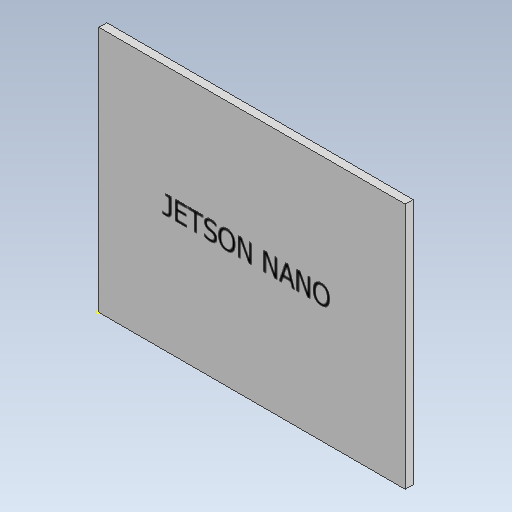
# Autodesk Inventor part: jetson_nano_sketch
Saved by Autodesk Inventor 2020 (Build 240168000, 168)
## iProperties
Created: 2019-10-22
Part Number: jetson_nano_sketch
Material: Generic
Document SubType Name: Modeling
Designer: Connor
Density: 1 g/cm^3
Appearance: Default
Author: Connor
Autodesk Inventor part; units mm, degrees
ref_plane "YZ Plane" through (0, 0, 0) normal (1, 0, 0) x (0, 1, 0)
ref_plane "XZ Plane" through (0, 0, 0) normal (0, 1, 0) x (-1, 0, 0)
ref_plane "XY Plane" through (0, 0, 0) normal (0, 0, 1) x (1, 0, 0)
sketch "Sketch1" plane through (0, 0, 0) normal (0, 0, 1) x (1, 0, 0)
  line L0 (0, 0) -> (0, 79.375)
  line L1 (0, 79.375) -> (98.425, 79.375)
  line L2 (98.425, 79.375) -> (98.425, 0)
  line L3 (98.425, 0) -> (0, 0)
  dimension "d0" = 79.375
  dimension "d1" = 98.425
  constraints: 8 end point, 3 perpendicular, 1 vertical
  measures "d0" distance of L0.start L0.end
  measures "d1" distance of L0.end L1.end
extrude "Extrusion1" add sketch "Sketch1" along normal blind 2.54
sketch "Sketch2" plane through (0, 0, 2.54) normal (0, 0, 1) x (1, 0, 0)
  line L0 (20.399, 43.9584) -> (88.2041, 43.9584) construction
  line L1 (88.2041, 43.9584) -> (88.2041, 3.4477) construction
  line L2 (88.2041, 3.4477) -> (20.399, 3.4477) construction
  line L3 (20.399, 3.4477) -> (20.399, 43.9584) construction
  point P0 (0, 0)
  constraints: 2 other
body "Solid1"
